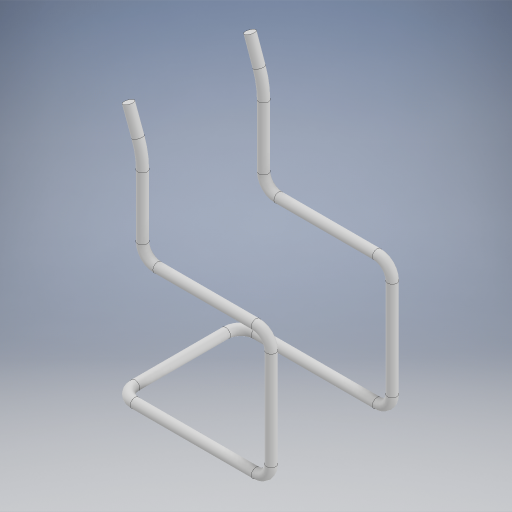
# Autodesk Inventor part: CE-1.4.1
Saved by Autodesk Inventor 2024 (Build 280153000, 153)
## iProperties
Created: 2024-01-25
Part Number: CE-1.4.1
Material: Generic
Document SubType Name: Modeling
Designer: Alex
Density: 1 g/cm^3
Appearance: Default
Author: Alex
Autodesk Inventor part; units mm, degrees
ref_plane "YZ Plane" through (0, 0, 0) normal (1, 0, 0) x (0, 1, 0)
ref_plane "XZ Plane" through (0, 0, 0) normal (0, 1, 0) x (-1, 0, 0)
ref_plane "Work Plane2" through (5.902, 170, -40.1492) normal (-0.342, 0.9397, -0.0056) x (-0.9397, -0.342, 0)
sketch "Sketch1" plane through (5.902, 170, -40.1492) normal (-0.342, 0.9397, -0.0056) x (-0.9397, -0.342, 0)
  circle A0 centre (0, 0) radius 3.175
  point P0 (63.6826, 39.2641)
  dimension "d18" = 6.35
  constraints: 1 centre point
  measures "d18" diameter of A0
sketch3d "3D Sketch1"
  line L0 (5.902, 170, -40.1492) -> (11.985, 153.2847, -40.0494)
  arc A0 (11.985, 153.2847, -40.0494) -> (15, 136.1837, -40) centre (-34.9933, 136.1837, -40.8197) ccw
  line L1 (15, 136.1837, -40) -> (15, 95, -40)
  arc A1 (15, 95, -40) -> (25, 85, -40) centre (25, 95, -40) ccw
  line L2 (25, 85, -40) -> (90, 85, -40)
  arc A2 (90, 85, -40) -> (100, 75, -40) centre (90, 75, -40) ccw
  line L3 (100, 75, -40) -> (100, 10, -40)
  arc A3 (100, 10, -40) -> (90, 0, -40) centre (90, 10, -40) ccw
  line L4 (90, 0, -40) -> (10, 0, -40)
  arc A4 (10, 0, -40) -> (0, 0, -30) centre (10, 0, -30) ccw
  line L5 (0, 0, -30) -> (0, 0, 0)
  line L6 (0, 0, 0) -> (0, 0, 30)
  arc A5 (0, 0, 30) -> (10, 0, 40) centre (10, 0, 30) ccw
  line L7 (10, 0, 40) -> (90, 0, 40)
  arc A6 (90, 0, 40) -> (100, 10, 40) centre (90, 10, 40) ccw
  line L8 (100, 10, 40) -> (100, 75, 40)
  arc A7 (100, 75, 40) -> (90, 85, 40) centre (90, 75, 40) ccw
  line L9 (90, 85, 40) -> (25, 85, 40)
  arc A8 (25, 85, 40) -> (15, 95, 40) centre (25, 95, 40) ccw
  line L10 (15, 95, 40) -> (15, 136.1837, 40)
  arc A9 (15, 136.1837, 40) -> (11.985, 153.2847, 40.0494) centre (-34.9933, 136.1837, 40.8197) ccw
  line L11 (11.985, 153.2847, 40.0494) -> (5.902, 170, 40.1492)
  dimension "d0" = 40
  dimension "d1" = 100
  dimension "d2" = 85
  dimension "d3" = 85
  dimension "d5" = 10
  dimension "d6" = 10
  dimension "d7" = 10
  dimension "d8" = 10
  dimension "d9" = 50
  dimension "d10" = 20
  dimension "d11" = 170
  dimension "d12" = 60
  dimension "d13" = 10
  dimension "d14" = 10
  dimension "d15" = 10
  dimension "d16" = 10
  dimension "d17" = 50
sweep "Sweep1" add profiles "Sketch1" path "3D Sketch1"
equation "\"d6\" = d5"
equation "\"d7\" = d5"
equation "\"d8\" = d5"
equation "\"d13\" = d5"
equation "\"d14\" = d6"
equation "\"d15\" = d7"
equation "\"d16\" = d8"
equation "\"d17\" = d9"
body "Solid1"
